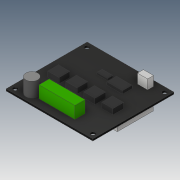
# Autodesk Inventor part: 모터드라이버
Saved by Autodesk Inventor 2018 (Build 220112000, 112)
## iProperties
Created: 2018-10-26
Part Number: 모터드라이버
Material: 일반
Document SubType Name: Modeling
Designer: dhksr
Density: 1 g/cm^3
Appearance: 기본값
Author: dhksr
Autodesk Inventor part; units mm, degrees
ref_plane "YZ Plane" through (0, 0, 0) normal (1, 0, 0) x (0, 1, 0)
ref_plane "XZ Plane" through (0, 0, 0) normal (0, 1, 0) x (-1, 0, 0)
ref_plane "XY Plane" through (0, 0, 0) normal (0, 0, 1) x (1, 0, 0)
sketch "스케치1" plane through (0, 0, 0) normal (0, 0, 1) x (1, 0, 0)
  line L0 (-36.25, -33.9) -> (36.25, -33.9)
  line L1 (36.25, -33.9) -> (36.25, 33.9)
  line L2 (36.25, 33.9) -> (-36.25, 33.9)
  line L3 (-36.25, 33.9) -> (-36.25, -33.9)
  line L4 (-36.25, -33.9) -> (36.25, 33.9) construction
  line L5 (36.25, -33.9) -> (-36.25, 33.9) construction
  line L6 (-32.5, -30) -> (32.5, -30) construction
  line L7 (32.5, -30) -> (32.5, 30) construction
  line L8 (32.5, 30) -> (-32.5, 30) construction
  line L9 (-32.5, 30) -> (-32.5, -30) construction
  line L10 (-32.5, -30) -> (32.5, 30) construction
  line L11 (32.5, -30) -> (-32.5, 30) construction
  circle A0 centre (-32.5, 30) radius 1.75
  circle A1 centre (-32.5, -30) radius 1.75
  line L12 (0, 0) -> (0, 9.9513)
  circle A2 centre (32.5, 30) radius 1.75
  circle A3 centre (32.5, -30) radius 1.75
  dimension "d0" = 72.5
  dimension "d1" = 67.8
  dimension "d2" = 65
  dimension "d3" = 60
  dimension "d4" = 3.5
  dimension "d5" = 3.5
  constraints: 26 end point, 4 centre point, 4 midpoint, 4 parallel, 2 coincident, 2 horizontal, 2 perpendicular, 2 symmetric about line, 1 vertical, 2 other
  measures "d0" distance of L2.end L1.end
  measures "d1" distance of L1.end L0.end
  measures "d2" distance of L8.end L7.end
  measures "d3" distance of L7.end L6.end
  measures "d4" diameter of A0
  measures "d5" diameter of A1
extrude "돌출1" add sketch "스케치1" along normal blind 1.55
sketch "스케치2" plane through (0, 0, 1.55) normal (0, 0, 1) x (1, 0, 0)
  circle A0 centre (32.5, -30) radius 1.75 projected
  circle A1 centre (-32.5, -30) radius 1.75 projected
  circle A2 centre (-32.5, 30) radius 1.75 projected
  line L0 (-36.25, -33.9) -> (36.25, -33.9) projected
  line L1 (36.25, -33.9) -> (36.25, 33.9) projected
  line L2 (36.25, 33.9) -> (-36.25, 33.9) projected
  line L3 (-15.25, -18.9) -> (14.75, -18.9)
  line L4 (14.75, -18.9) -> (14.75, -27.4)
  line L5 (14.75, -27.4) -> (-15.25, -27.4)
  line L6 (-15.25, -27.4) -> (-15.25, -18.9)
  line L7 (-27.25, 0.9) -> (-17.75, 0.9)
  line L8 (-17.75, 0.9) -> (-17.75, -8.1)
  line L9 (-17.75, -8.1) -> (-27.25, -8.1)
  line L10 (-27.25, -8.1) -> (-27.25, 0.9)
  line L11 (-12.25, 0.9) -> (-2.75, 0.9)
  line L12 (-2.75, 0.9) -> (-2.75, -8.1)
  line L13 (-2.75, -8.1) -> (-12.25, -8.1)
  line L14 (-12.25, -8.1) -> (-12.25, 0.9)
  line L15 (3.25, 18.9) -> (16.25, 18.9)
  line L16 (16.25, 18.9) -> (16.25, 10.9)
  line L17 (16.25, 10.9) -> (3.25, 10.9)
  line L18 (3.25, 10.9) -> (3.25, 18.9)
  circle A3 centre (-22.25, -26.4) radius 5
  line L19 (-8.75, 18.9) -> (0.25, 18.9)
  line L20 (0.25, 18.9) -> (0.25, 14.4)
  line L21 (0.25, 14.4) -> (-8.75, 14.4)
  line L22 (-8.75, 14.4) -> (-8.75, 18.9)
  line L23 (15.25, 29.4) -> (23.75, 29.4)
  line L24 (23.75, 29.4) -> (23.75, 24.4)
  line L25 (23.75, 24.4) -> (15.25, 24.4)
  line L26 (15.25, 24.4) -> (15.25, 29.4)
  point P0 (0, 0)
  dimension "d8" = 10
  dimension "d9" = 8.5
  dimension "d10" = 30
  dimension "d11" = 9
  dimension "d12" = 9.5
  dimension "d13" = 9.5
  dimension "d14" = 13
  dimension "d15" = 8
  dimension "d20" = 6.5
  dimension "d21" = 21.5
  dimension "d23" = 5.5
  dimension "d24" = 33
  dimension "d25" = 10
  dimension "d26" = 20
  dimension "d27" = 9
  dimension "d28" = 4.5
  dimension "d29" = 3
  dimension "d30" = 15
  dimension "d32" = 8.5
  dimension "d33" = 5
  dimension "d34" = 12.5
  dimension "d35" = 4.5
  dimension "d36" = 2.5
  dimension "d38" = 65
  dimension "d39" = 60
  constraints: 48 end point, 12 parallel, 6 horizontal, 6 perpendicular, 2 point on line, 1 centre point
  measures "d8" diameter of A3
  measures "d9" distance of L5.end L3.start
  measures "d10" distance of L3.start L3.end
  measures "d11" distance of L11.end L12.end
  measures "d12" distance of L11.start L11.end
  measures "d13" distance of L7.start L7.end
  measures "d14" distance of L15.start L15.end
  measures "d15" distance of L15.end L16.end
  measures "d20" distance between parallel lines of L0 L5
  measures "d21" distance between parallel lines of L1 L4
  measures "d23" distance between parallel lines of L14 L8
  measures "d24" distance between parallel lines of L2 L7
  measures "d25" distance between parallel lines of L17 L11
  measures "d26" distance between parallel lines of L1 L16
  measures "d27" distance of L20.end L21.end
  measures "d28" distance of L19.end L20.end
  measures "d29" distance between parallel lines of L18 L20
  measures "d30" distance between parallel lines of L2 L19
  measures "d32" distance of L24.end L25.end
  measures "d33" distance of L23.end L24.end
  measures "d34" distance between parallel lines of L1 L24
  measures "d35" distance between parallel lines of L2 L23
  measures "d36" distance edge to line of A3 L0
  measures "d38" distance of A0.centre A1.centre
  measures "d39" distance of A1.centre A2.centre
extrude "돌출2" add sketch "스케치2" along normal blind 12.2 contours A3
extrude "돌출3" add sketch "스케치2" along normal blind 4.5 contours L7 L8 L9 L10 | L11 L12 L13 L14
extrude "돌출4" add sketch "스케치2" along normal blind 10.2 contours L3 L4 L5 L6
extrude "돌출5" add sketch "스케치2" along normal blind 2.5 contours L15 L16 L17 L18
extrude "돌출6" add sketch "스케치2" along normal blind 1.5 contours L19 L20 L21 L22
extrude "돌출7" add sketch "스케치2" along normal blind 8 contours L23 L24 L25 L26
mirror "미러1" about plane through (0, 0, 0) normal (1, 0, 0) of "돌출3"
sketch "스케치4" plane through (0, 0, 0) normal (0, 0, -1) x (-1, 0, 0)
  line L0 (-36.25, -33.9) -> (-36.25, 33.9) projected
  line L1 (-29.75, 23.1) -> (-29.75, -6.9)
  line L2 (-29.75, -6.9) -> (29.75, -6.9)
  line L3 (29.75, -6.9) -> (29.75, 23.1)
  line L4 (29.75, 23.1) -> (-29.75, 23.1)
  line L5 (36.25, -33.9) -> (-36.25, -33.9) projected
  point P0 (0, 0)
  point P1 (0, 23.1)
  point P2 (-36.25, 0)
  dimension "d53" = 59.5
  dimension "d54" = 30
  dimension "d58" = 27
  constraints: 8 end point, 2 midpoint, 2 parallel, 1 perpendicular
  measures "d53" distance of L3.end L1.start
  measures "d54" distance of L2.end L3.end
  measures "d58" distance between parallel lines of L5 L2
extrude "돌출8" add sketch "스케치4" along normal blind 10
